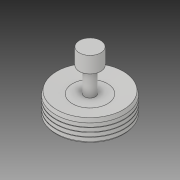
# Autodesk Inventor part: Top1
Saved by Autodesk Inventor 2018 (Build 220112000, 112)
## iProperties
Created: 2017-12-12
Part Number: Top1
Material: Generic
Document SubType Name: Modeling
Designer: Rus
Density: 1 g/cm^3
Appearance: Default
Author: Rus
Autodesk Inventor part; units mm, degrees
ref_plane "YZ Plane" through (0, 0, 0) normal (1, 0, 0) x (0, 1, 0)
ref_plane "XZ Plane" through (0, 0, 0) normal (0, 1, 0) x (-1, 0, 0)
ref_plane "XY Plane" through (0, 0, 0) normal (0, 0, 1) x (1, 0, 0)
sketch "Sketch1" plane through (0, 0, 0) normal (0, 0, 1) x (1, 0, 0)
  line L0 (0, 0) -> (0, 28.575)
  line L1 (0, 0) -> (0, -6.35)
  line L2 (0, 28.575) -> (0, 38.1)
  line L3 (6.35, 28.575) -> (6.35, 38.1)
  line L4 (6.35, 38.1) -> (0, 38.1)
  line L5 (3.175, 17.0324) -> (0, 17.0324) construction
  line L6 (6.35, 28.575) -> (3.175, 28.575)
  line L7 (3.175, 28.575) -> (0, 28.575) construction
  line L8 (0, 0) -> (3.175, 0) construction
  line L9 (3.175, 0) -> (3.175, 0) construction
  line L10 (19.7047, 2.9146) -> (20.32, 3.7934)
  line L11 (0, -6.35) -> (3.175, -4.2333)
  line L12 (3.175, -4.2333) -> (3.175, 0)
  line L13 (3.175, 0) -> (19.7047, 2.9146)
  line L14 (3.175, 28.575) -> (3.175, 13.97)
  line L15 (20.32, 8.7146) -> (20.1613, 8.5559) construction
  line L16 (20.1613, 8.5559) -> (20.32, 8.3971) construction
  arc A0 (6.35, 38.1) -> (0, 40.0262) centre (0, 28.5962) ccw
  line L17 (20.32, 6.254) -> (20.1613, 6.0952) construction
  line L18 (20.1613, 6.0952) -> (20.32, 5.9365) construction
  line L19 (20.32, 10.8577) -> (20.1613, 11.0165) construction
  line L20 (20.1613, 11.0165) -> (20.32, 11.1752) construction
  line L21 (20.32, 3.7934) -> (20.32, 5.9365)
  line L22 (20.32, 6.254) -> (20.32, 8.3971)
  line L23 (20.32, 8.7146) -> (20.32, 10.8577)
  line L24 (20.32, 11.1752) -> (20.32, 13.3184)
  line L25 (20.32, 5.9365) -> (20.32, 6.254) construction
  line L26 (20.32, 8.3971) -> (20.32, 8.7146) construction
  line L27 (20.32, 10.8577) -> (20.32, 11.1752) construction
  arc A1 (20.32, 11.1752) -> (20.32, 10.8577) centre (20.4787, 11.0165) ccw
  arc A2 (20.32, 8.7146) -> (20.32, 8.3971) centre (20.4787, 8.5559) ccw
  arc A3 (20.32, 6.254) -> (20.32, 5.9365) centre (20.4787, 6.0952) ccw
  line L28 (20.1613, 8.5559) -> (0, 8.5559) construction
  line L29 (19.7047, 15.6146) -> (10.3775, 13.97)
  line L30 (20.32, 13.3184) -> (19.7047, 15.6146)
  line L31 (3.175, 12.7) -> (3.175, 13.97) construction
  line L32 (3.175, 13.97) -> (10.3775, 13.97)
  line L33 (10.3775, 13.97) -> (3.175, 12.7) construction
  line L34 (3.175, 13.97) -> (3.175, 12.7) construction
  dimension "d5" = 44.45
  dimension "d6" = 9.525
  dimension "d7" = 6.35
  dimension "d12" = 2.1167
  dimension "d13" = 3.175
  dimension "d15" = 4.2333
  dimension "d24" = 10
  dimension "d28" = 3.175
  dimension "d36" = 0.3175
  dimension "d37" = 9.525
  dimension "d40" = 11.43
  dimension "d42" = 20.32
  dimension "d43" = 55
  dimension "d45" = 15.875
  dimension "d46" = 75
  dimension "d47" = 1.27
  constraints: 71 end point, 12 vertical, 8 equal length, 8 point on circle, 5 perpendicular, 5 point on line, 4 centre point, 4 horizontal, 3 collinear, 3 parallel, 2 equal radius, 1 line through centre, 1 tangent, 1 vertical alignment
  measures "d5" distance of L2.end L1.end
  measures "d6" distance of L3.start L3.end
  measures "d7" distance between parallel lines of L2 L3
  measures "d12" vertical distance of L11.end L1.end
  measures "d13" horizontal distance of L1.end L11.end
  measures "d15" distance from line of L9 L11.end
  measures "d24" angle of L13 L9
  measures "d28" distance of L3.start L6.end
  measures "d36" distance of L15.start L16.end
  measures "d37" distance of L24.end L10.end
  measures "d40" radius of A0
  measures "d42" distance between parallel lines of L22 L0
  measures "d43" angle of L28 L10
  measures "d45" distance of L6.end L31.start
  measures "d46" angle of L28 L30
  measures "d47" distance of L31.start L14.end
revolve "Revolution1" add sketch "Sketch1" angle 360 about axis through (0, 28.575, 0) along (0, -1, 0)
body "Solid1"
